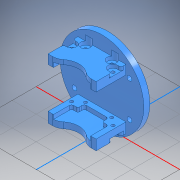
# Autodesk Inventor part: 000.005.005.001 - ОСНОВАНИЕ
Saved by Autodesk Inventor 2022 (Build 260153000, 153)
## iProperties
Created: 2022-12-19
Part Number: 000.005.005.001 - ОСНОВАНИЕ
Material: Пластик АБС
Document SubType Name: Modeling
Designer: Ivan Petrov
Density: 1.06 g/cm^3
Appearance: Голубой
Author: Ivan Petrov
Autodesk Inventor part; units mm, degrees
ref_plane "YZ Plane" through (0, 0, 0) normal (1, 0, 0) x (0, 1, 0)
ref_plane "XZ Plane" through (0, 0, 0) normal (0, 1, 0) x (-1, 0, 0)
ref_plane "XY Plane" through (0, 0, 0) normal (0, 0, 1) x (1, 0, 0)
sketch "Эскиз1" plane through (0, 0, 0) normal (0, 0, 1) x (1, 0, 0)
  circle A0 centre (0, 0) radius 35
  dimension "d7" = 70
  constraints: 1 centre point
  measures "d7" diameter of A0
sketch "Эскиз1 outline for Выдавливание1" plane through (0, 0, 0) normal (0, 0, 1) x (1, 0, 0)
  circle A0 centre (0, 0) radius 35
extrude "Выдавливание1" add sketch "Эскиз1 outline for Выдавливание1" along normal blind 5
sketch "Эскиз2" plane through (0, 0, 5) normal (0, 0, 1) x (1, 0, 0)
  circle A0 centre (-23, 15) radius 2
  point P0 (0, 0)
  dimension "d4" = 4
  dimension "d5" = 15
  dimension "d6" = 23
  constraints: 1 centre point
  measures "d4" diameter of A0
  measures "d5" vertical distance of A0.centre point (0, 0)
  measures "d6" horizontal distance of point (0, 0) A0.centre
sketch "Эскиз2 outline for Выдавливание2" plane through (0, 0, 5) normal (0, 0, 1) x (1, 0, 0)
  circle A0 centre (-23, 15) radius 2
extrude "Выдавливание2" cut sketch "Эскиз2 outline for Выдавливание2" against normal through all
mirror "Зеркальное отражение1" about plane through (0, 0, 0) normal (0, 1, 0) of "Выдавливание2"
mirror "Зеркальное отражение2" about plane through (0, 0, 0) normal (1, 0, 0) of "Выдавливание2", "Зеркальное отражение1"
sketch "Эскиз9" plane through (0, 0, 5) normal (0, 0, 1) x (1, 0, 0)
  line L0 (20.1, 16) -> (20.1, 13.5) projected
  line L1 (-20.1, 16) -> (-20.1, 13.5) projected
  line L2 (20.1, 16) -> (-20.1, 16)
  line L3 (-20.1, 16) -> (-20.1, 18.6)
  line L4 (-20.1, 18.6) -> (20.1, 18.6)
  line L5 (20.1, 18.6) -> (20.1, 16)
  line L6 (-13, 18.6) -> (13, 18.6)
  point P0 (0, 0)
  constraints: 10 end point, 2 horizontal, 2 parallel, 1 perpendicular, 1 point on line, 2 other
sketch "Эскиз9 outline for Выдавливание8" plane through (0, 0, 5) normal (0, 0, 1) x (1, 0, 0)
  line L0 (-20.1, 18.6) -> (-20.1, 16)
  line L1 (20.1, 18.6) -> (-20.1, 18.6)
  line L2 (20.1, 16) -> (20.1, 18.6)
  line L3 (-20.1, 16) -> (20.1, 16)
extrude "Выдавливание8" add sketch "Эскиз9 outline for Выдавливание8" along normal blind 25
sketch "Эскиз10" plane through (0, 0, 5) normal (0, 0, 1) x (1, 0, 0)
  line L0 (20.1, -15.5) -> (20.1, -18)
  line L1 (-20.1, -15.5) -> (-20.1, -18)
  line L2 (20.1, -18) -> (-20.1, -18)
  line L3 (-20.1, -18) -> (-20.1, -21.499996)
  line L4 (-20.1, -21.499996) -> (20.1, -21.499996)
  line L5 (20.1, -21.499996) -> (20.1, -18)
  line L6 (7.682609, -21.499996) -> (-7.682606, -21.5)
  point P0 (0, 0)
  constraints: 8 end point, 2 parallel, 1 horizontal, 1 perpendicular, 1 point on line
sketch "Эскиз10 outline for Выдавливание9" plane through (0, 0, 5) normal (0, 0, 1) x (1, 0, 0)
  line L0 (20.1, -21.499996) -> (20.1, -18)
  line L1 (-20.1, -21.499996) -> (20.1, -21.499996)
  line L2 (-20.1, -18) -> (-20.1, -21.499996)
  line L3 (20.1, -18) -> (-20.1, -18)
extrude "Выдавливание9" add sketch "Эскиз10 outline for Выдавливание9" along normal blind 25
sketch "Эскиз11" plane through (-20.1, 18.6, 5) normal (0, 1, 0) x (1, 0, 0)
  arc A0 (0, -52.676629) -> (0.51922, -54.36356) centre (3, -52.676629) ccw
  line L0 (0.51922, -54.36356) -> (4.504742, -60.22462)
  arc A1 (4.504742, -60.22462) -> (6.158595, -61.1) centre (6.158595, -59.1) ccw
  line L1 (7.1, -61.1) -> (6.158595, -61.1)
  arc A2 (5.6, -59.6) -> (7.1, -61.1) centre (7.1, -59.6) ccw
  line L2 (5.6, -6.6) -> (5.6, -59.6)
  arc A3 (6.6, -5.6) -> (5.6, -6.6) centre (6.6, -6.6) ccw
  line L3 (33.6, -5.6) -> (6.6, -5.6)
  arc A4 (34.6, -6.6) -> (33.6, -5.6) centre (33.6, -6.6) ccw
  line L4 (34.6, -59.6) -> (34.6, -6.6)
  arc A5 (33.1, -61.1) -> (34.6, -59.6) centre (33.1, -59.6) ccw
  line L5 (34.041405, -61.1) -> (33.1, -61.1)
  arc A6 (34.041405, -61.1) -> (35.695258, -60.22462) centre (34.041405, -59.1) ccw
  line L6 (35.695258, -60.22462) -> (39.68078, -54.36356)
  arc A7 (39.68078, -54.36356) -> (40.2, -52.676629) centre (37.2, -52.676629) ccw
  line L7 (40.2, -52.676629) -> (40.2, -8.423371)
  arc A8 (40.2, -8.423371) -> (39.68078, -6.73644) centre (37.2, -8.423371) ccw
  line L8 (39.68078, -6.73644) -> (35.992888, -1.31307)
  arc A9 (35.992888, -1.31307) -> (33.512108, 0) centre (33.512108, -3) ccw
  line L9 (33.512108, 0) -> (6.687892, 0)
  arc A10 (6.687892, 0) -> (4.207112, -1.31307) centre (6.687892, -3) ccw
  line L10 (4.207112, -1.31307) -> (0.51922, -6.73644)
  arc A11 (0.51922, -6.73644) -> (0, -8.423371) centre (3, -8.423371) ccw
  line L11 (0, -8.423371) -> (0, -52.676629)
  circle A12 centre (37.4, -52.1) radius 1.35
  circle A13 centre (37.4, -30.1) radius 1.35
  circle A14 centre (31.1, -2.8) radius 1.35
  circle A15 centre (2.8, -52.1) radius 1.35
  circle A16 centre (2.8, -30.1) radius 1.35
  circle A17 centre (9.1, -2.8) radius 1.35
  circle A18 centre (37.4, -8.1) radius 1.35
  circle A19 centre (2.8, -8.1) radius 1.35
  line L12 (7.1, -61.1) -> (33.1, -61.1)
  point P0 (20.1, 5)
  point P1 (20.1, -48.1)
  point P2 (20.1, -48.1)
  constraints: 26 end point, 24 point on circle, 20 centre point
sketch "Эскиз11 outline for Выдавливание10" plane through (-20.1, 18.6, 5) normal (0, 1, 0) x (1, 0, 0)
  circle A0 centre (2.8, -8.1) radius 1.35
  circle A1 centre (9.1, -2.8) radius 1.35
  circle A2 centre (31.1, -2.8) radius 1.35
  circle A3 centre (37.4, -8.1) radius 1.35
extrude "Выдавливание10" cut sketch "Эскиз11 outline for Выдавливание10" against normal through all
sketch "Эскиз12" plane through (-20.1, 18.6, 5) normal (0, 1, 0) x (1, 0, 0)
  arc A0 (0, -52.676629) -> (0.51922, -54.36356) centre (3, -52.676629) ccw
  line L0 (0.51922, -54.36356) -> (4.504742, -60.22462)
  arc A1 (4.504742, -60.22462) -> (6.158595, -61.1) centre (6.158595, -59.1) ccw
  line L1 (7.1, -61.1) -> (6.158595, -61.1)
  arc A2 (5.6, -59.6) -> (7.1, -61.1) centre (7.1, -59.6) ccw
  line L2 (5.6, -6.6) -> (5.6, -59.6)
  arc A3 (6.6, -5.6) -> (5.6, -6.6) centre (6.6, -6.6) ccw
  line L3 (33.6, -5.6) -> (6.6, -5.6)
  arc A4 (34.6, -6.6) -> (33.6, -5.6) centre (33.6, -6.6) ccw
  line L4 (34.6, -59.6) -> (34.6, -6.6)
  arc A5 (33.1, -61.1) -> (34.6, -59.6) centre (33.1, -59.6) ccw
  line L5 (34.041405, -61.1) -> (33.1, -61.1)
  arc A6 (34.041405, -61.1) -> (35.695258, -60.22462) centre (34.041405, -59.1) ccw
  line L6 (35.695258, -60.22462) -> (39.68078, -54.36356)
  arc A7 (39.68078, -54.36356) -> (40.2, -52.676629) centre (37.2, -52.676629) ccw
  line L7 (40.2, -52.676629) -> (40.2, -8.423371)
  arc A8 (40.2, -8.423371) -> (39.68078, -6.73644) centre (37.2, -8.423371) ccw
  line L8 (39.68078, -6.73644) -> (35.992888, -1.31307)
  arc A9 (35.992888, -1.31307) -> (33.512108, 0) centre (33.512108, -3) ccw
  line L9 (33.512108, 0) -> (6.687892, 0)
  arc A10 (6.687892, 0) -> (4.207112, -1.31307) centre (6.687892, -3) ccw
  line L10 (4.207112, -1.31307) -> (0.51922, -6.73644)
  arc A11 (0.51922, -6.73644) -> (0, -8.423371) centre (3, -8.423371) ccw
  line L11 (0, -8.423371) -> (0, -52.676629)
  circle A12 centre (37.4, -52.1) radius 1.35
  circle A13 centre (37.4, -30.1) radius 1.35
  circle A14 centre (31.1, -2.8) radius 1.35
  circle A15 centre (2.8, -52.1) radius 1.35
  circle A16 centre (2.8, -30.1) radius 1.35
  circle A17 centre (9.1, -2.8) radius 1.35
  circle A18 centre (37.4, -8.1) radius 1.35
  circle A19 centre (2.8, -8.1) radius 1.35
  line L12 (7.1, -61.1) -> (33.1, -61.1)
  point P0 (20.1, 5)
  point P1 (20.1, 5)
  point P2 (20.1, -48.1)
  point P3 (20.1, -48.1)
  constraints: 26 end point, 24 point on circle, 20 centre point
sketch "Эскиз12 outline for Выдавливание11" plane through (-20.1, 18.6, 5) normal (0, 1, 0) x (1, 0, 0)
  line L0 (34.6, -59.6) -> (34.6, -6.6)
  arc A0 (33.1, -61.1) -> (34.6, -59.6) centre (33.1, -59.6) ccw
  line L1 (7.1, -61.1) -> (33.1, -61.1)
  arc A1 (5.6, -59.6) -> (7.1, -61.1) centre (7.1, -59.6) ccw
  line L2 (5.6, -6.6) -> (5.6, -59.6)
  arc A2 (6.6, -5.6) -> (5.6, -6.6) centre (6.6, -6.6) ccw
  line L3 (33.6, -5.6) -> (6.6, -5.6)
  arc A3 (34.6, -6.6) -> (33.6, -5.6) centre (33.6, -6.6) ccw
extrude "Выдавливание11" cut sketch "Эскиз12 outline for Выдавливание11" against normal blind 10
sketch "Эскиз13" plane through (-20.1, -21.499996, 5) normal (0, -1, 0) x (1, 0, 0)
  arc A0 (0.51922, 54.36356) -> (0, 52.676629) centre (3, 52.676629) ccw
  line L0 (0, 8.423371) -> (0, 52.676629)
  arc A1 (0, 8.423371) -> (0.51922, 6.73644) centre (3, 8.423371) ccw
  line L1 (4.207112, 1.31307) -> (0.51922, 6.73644)
  arc A2 (4.207112, 1.31307) -> (6.687892, 0) centre (6.687892, 3) ccw
  line L2 (33.512108, 0) -> (6.687892, 0)
  arc A3 (33.512108, 0) -> (35.992888, 1.31307) centre (33.512108, 3) ccw
  line L3 (39.68078, 6.73644) -> (35.992888, 1.31307)
  arc A4 (39.68078, 6.73644) -> (40.2, 8.423371) centre (37.2, 8.423371) ccw
  line L4 (40.2, 52.676629) -> (40.2, 8.423371)
  arc A5 (40.2, 52.676629) -> (39.68078, 54.36356) centre (37.2, 52.676629) ccw
  line L5 (35.695258, 60.22462) -> (39.68078, 54.36356)
  arc A6 (35.695258, 60.22462) -> (34.041405, 61.1) centre (34.041405, 59.1) ccw
  line L6 (27.75, 61.1) -> (34.041405, 61.1)
  arc A7 (29.25, 59.6) -> (27.75, 61.1) centre (27.75, 59.6) ccw
  line L7 (29.25, 59.6) -> (29.25, 58.1)
  arc A8 (29.25, 58.1) -> (31.6, 55.75) centre (31.6, 58.1) ccw
  line L8 (31.6, 55.75) -> (33.6, 55.75)
  arc A9 (34.6, 54.75) -> (33.6, 55.75) centre (33.6, 54.75) ccw
  line L9 (34.6, 54.75) -> (34.6, 11.95)
  arc A10 (33.6, 10.95) -> (34.6, 11.95) centre (33.6, 11.95) ccw
  line L10 (33.6, 10.95) -> (31.6, 10.95)
  arc A11 (31.6, 10.95) -> (29.25, 8.6) centre (31.6, 8.6) ccw
  line L11 (29.25, 8.6) -> (29.25, 6.6)
  arc A12 (28.25, 5.6) -> (29.25, 6.6) centre (28.25, 6.6) ccw
  line L12 (28.25, 5.6) -> (11.95, 5.6)
  arc A13 (10.95, 6.6) -> (11.95, 5.6) centre (11.95, 6.6) ccw
  line L13 (10.95, 6.6) -> (10.95, 8.6)
  arc A14 (10.95, 8.6) -> (8.6, 10.95) centre (8.6, 8.6) ccw
  line L14 (8.6, 10.95) -> (6.6, 10.95)
  arc A15 (5.6, 11.95) -> (6.6, 10.95) centre (6.6, 11.95) ccw
  line L15 (5.6, 11.95) -> (5.6, 54.75)
  arc A16 (6.6, 55.75) -> (5.6, 54.75) centre (6.6, 54.75) ccw
  line L16 (6.6, 55.75) -> (8.6, 55.75)
  arc A17 (8.6, 55.75) -> (10.95, 58.1) centre (8.6, 58.1) ccw
  line L17 (10.95, 58.1) -> (10.95, 59.6)
  arc A18 (12.45, 61.1) -> (10.95, 59.6) centre (12.45, 59.6) ccw
  line L18 (6.158595, 61.1) -> (12.45, 61.1)
  arc A19 (6.158595, 61.1) -> (4.504742, 60.22462) centre (6.158595, 59.1) ccw
  line L19 (0.51922, 54.36356) -> (4.504742, 60.22462)
  circle A20 centre (37.4, 52.1) radius 1.35
  circle A21 centre (37.4, 30.1) radius 1.35
  circle A22 centre (31.1, 2.8) radius 1.35
  circle A23 centre (2.8, 52.1) radius 1.35
  circle A24 centre (2.8, 30.1) radius 1.35
  circle A25 centre (9.1, 2.8) radius 1.35
  circle A26 centre (37.4, 8.1) radius 1.35
  circle A27 centre (2.8, 8.1) radius 1.35
  circle A28 centre (20.1, 48.1) radius 1.6
  line L20 (12.45, 61.1) -> (27.75, 61.1)
  point P0 (20.1, -5)
  constraints: 42 end point, 40 point on circle, 28 centre point, 1 horizontal
sketch "Эскиз13 outline for Выдавливание12" plane through (-20.1, -21.499996, 5) normal (0, -1, 0) x (1, 0, 0)
  arc A0 (12.45, 61.1) -> (10.95, 59.6) centre (12.45, 59.6) ccw
  line L0 (27.75, 61.1) -> (12.45, 61.1)
  line L1 (10.95, 59.6) -> (10.95, 58.1)
  arc A1 (29.25, 59.6) -> (27.75, 61.1) centre (27.75, 59.6) ccw
  arc A2 (10.95, 58.1) -> (8.6, 55.75) centre (8.6, 58.1) cw
  line L2 (29.25, 58.1) -> (29.25, 59.6)
  line L3 (8.6, 55.75) -> (6.6, 55.75)
  arc A3 (31.6, 55.75) -> (29.25, 58.1) centre (31.6, 58.1) cw
  arc A4 (6.6, 55.75) -> (5.6, 54.75) centre (6.6, 54.75) ccw
  line L4 (33.6, 55.75) -> (31.6, 55.75)
  line L5 (5.6, 54.75) -> (5.6, 11.95)
  arc A5 (34.6, 54.75) -> (33.6, 55.75) centre (33.6, 54.75) ccw
  arc A6 (5.6, 11.95) -> (6.6, 10.95) centre (6.6, 11.95) ccw
  line L6 (34.6, 11.95) -> (34.6, 54.75)
  line L7 (6.6, 10.95) -> (8.6, 10.95)
  arc A7 (33.6, 10.95) -> (34.6, 11.95) centre (33.6, 11.95) ccw
  arc A8 (8.6, 10.95) -> (10.95, 8.6) centre (8.6, 8.6) cw
  line L8 (31.6, 10.95) -> (33.6, 10.95)
  line L9 (10.95, 8.6) -> (10.95, 6.6)
  arc A9 (29.25, 8.6) -> (31.6, 10.95) centre (31.6, 8.6) cw
  arc A10 (10.95, 6.6) -> (11.95, 5.6) centre (11.95, 6.6) ccw
  line L10 (29.25, 6.6) -> (29.25, 8.6)
  line L11 (11.95, 5.6) -> (28.25, 5.6)
  arc A11 (28.25, 5.6) -> (29.25, 6.6) centre (28.25, 6.6) ccw
  circle A12 centre (20.1, 48.1) radius 1.6
extrude "Выдавливание12" cut sketch "Эскиз13 outline for Выдавливание12" against normal blind 10
offset faces "Размер5" outward -1 faces at (-14.5, 17.733333, 17.733333) (-14.455573, 17.733333, 11.305245) (4.5, 17.733333, 10.6) (14.430874, 16.866667, 11.234659) (14.5, 17.733333, 23.866667) (-2.716667, -20.333331, 10.6) (8.22473, -20.333331, 10.602796) (9.176248, -19.166665, 13.950249) (9.15, -20.333331, 12.266667) (12.166667, -20.333331, 15.95) (14.488831, -19.166665, 16.800958) (14.5, -19.166665, 21.3) (-9.138831, -19.166665, 11.450958) (-9.15, -20.333331, 12.933333) (-11.149751, -19.166665, 15.923752) (-12.833333, -19.166665, 15.95) (-14.180173, -19.166665, 16.216948) (-14.5, -20.333331, 25.65)
sketch "Эскиз14" plane through (-20.1, -21.499996, 5) normal (0, -1, 0) x (1, 0, 0)
  line L0 (35.6, 25) -> (35.6, 11.95) projected
  arc A0 (33.6, 9.95) -> (35.6, 11.95) centre (33.6, 11.95) ccw projected
  line L1 (33.6, 9.95) -> (31.6, 9.95) projected
  arc A1 (31.6, 9.95) -> (30.25, 8.6) centre (31.6, 8.6) ccw projected
  line L2 (30.25, 8.6) -> (30.25, 6.6) projected
  arc A2 (28.25, 4.6) -> (30.25, 6.6) centre (28.25, 6.6) ccw projected
  line L3 (28.25, 4.6) -> (11.95, 4.6) projected
  arc A3 (9.95, 6.6) -> (11.95, 4.6) centre (11.95, 6.6) ccw projected
  line L4 (9.95, 6.6) -> (9.95, 8.6) projected
  arc A4 (9.95, 8.6) -> (8.6, 9.95) centre (8.6, 8.6) ccw projected
  line L5 (8.6, 9.95) -> (6.6, 9.95) projected
  arc A5 (4.6, 11.95) -> (6.6, 9.95) centre (6.6, 11.95) ccw projected
  line L6 (4.6, 11.95) -> (4.6, 25) projected
  line L7 (0, 25) -> (4.6, 25) projected
  line L8 (0, 0) -> (0, 25) projected
  line L9 (40.2, 0) -> (0, 0) projected
  line L10 (40.2, 0) -> (40.2, 25) projected
  line L11 (35.6, 25) -> (40.2, 25) projected
  circle A6 centre (37.4, 8.1) radius 1.35 projected
  circle A7 centre (2.8, 8.1) radius 1.35 projected
  circle A8 centre (31.1, 2.8) radius 1.35 projected
  circle A9 centre (9.1, 2.8) radius 1.35 projected
  line L12 (4.6, 6.6) -> (4.6, 25) projected
  line L13 (4.6, 25) -> (36.05, 25)
  point P0 (20.1, -5)
  constraints: 2 end point, 1 point on line
sketch "Эскиз14 outline for Выдавливание13" plane through (-20.1, -21.499996, 5) normal (0, -1, 0) x (1, 0, 0)
  line L0 (4.6, 25) -> (0, 25)
  line L1 (35.6, 25) -> (4.6, 25)
  line L2 (0, 25) -> (0, 0)
  line L3 (40.2, 25) -> (35.6, 25)
  line L4 (0, 0) -> (40.2, 0)
  line L5 (40.2, 0) -> (40.2, 25)
  circle A0 centre (9.1, 2.8) radius 1.35
  circle A1 centre (31.1, 2.8) radius 1.35
  circle A2 centre (2.8, 8.1) radius 1.35
  circle A3 centre (37.4, 8.1) radius 1.35
extrude "Выдавливание13" add sketch "Эскиз14 outline for Выдавливание13" along normal blind 5
sketch "Эскиз15" plane through (-20.1, 18.6, 5) normal (0, 1, 0) x (1, 0, 0)
  line L0 (4.6, -25) -> (4.6, -6.6) projected
  arc A0 (6.6, -4.6) -> (4.6, -6.6) centre (6.6, -6.6) ccw projected
  line L1 (6.6, -4.6) -> (33.6, -4.6) projected
  arc A1 (35.6, -6.6) -> (33.6, -4.6) centre (33.6, -6.6) ccw projected
  line L2 (35.6, -6.6) -> (35.6, -25) projected
  line L3 (40.2, -25) -> (35.6, -25) projected
  line L4 (40.2, 0) -> (40.2, -25) projected
  line L5 (0, 0) -> (40.2, 0) projected
  line L6 (0, 0) -> (0, -25) projected
  line L7 (4.6, -25) -> (0, -25) projected
  circle A2 centre (37.4, -8.1) radius 1.35 projected
  circle A3 centre (2.8, -8.1) radius 1.35 projected
  circle A4 centre (31.1, -2.8) radius 1.35 projected
  circle A5 centre (9.1, -2.8) radius 1.35 projected
  line L8 (35.6, -25) -> (4.6, -25)
  line L9 (40.2, -25) -> (0, -25) projected
  point P0 (20.1, 5)
  constraints: 2 end point, 1 collinear
sketch "Эскиз15 outline for Выдавливание14" plane through (-20.1, 18.6, 5) normal (0, 1, 0) x (1, 0, 0)
  line L0 (4.6, -25) -> (35.6, -25)
  line L1 (0, -25) -> (4.6, -25)
  line L2 (35.6, -25) -> (40.2, -25)
  line L3 (0, 0) -> (0, -25)
  line L4 (40.2, -25) -> (40.2, 0)
  line L5 (40.2, 0) -> (0, 0)
  circle A0 centre (2.8, -8.1) radius 1.35
  circle A1 centre (37.4, -8.1) radius 1.35
  circle A2 centre (9.1, -2.8) radius 1.35
  circle A3 centre (31.1, -2.8) radius 1.35
extrude "Выдавливание14" add sketch "Эскиз15 outline for Выдавливание14" along normal blind 5
sketch "Эскиз16" plane through (-20.1, 23.6, 5) normal (0, 1, 0) x (1, 0, 0)
  circle A0 centre (37.4, -8.1) radius 1.35 projected
  circle A1 centre (37.4, -8.1) radius 4
  circle A2 centre (31.1, -2.8) radius 1.35 projected
  circle A3 centre (31.1, -2.8) radius 4
  circle A4 centre (2.8, -8.1) radius 1.35 projected
  circle A5 centre (2.8, -8.1) radius 4
  circle A6 centre (9.1, -2.8) radius 1.35 projected
  circle A7 centre (9.1, -2.8) radius 4
  point P0 (20.1, 5)
  dimension "d51" = 8
  dimension "d52" = 8
  dimension "d53" = 8
  dimension "d54" = 8
  constraints: 4 centre point, 4 coincident
  measures "d51" diameter of A1
  measures "d52" diameter of A3
  measures "d53" diameter of A5
  measures "d54" diameter of A7
sketch "Эскиз16 outline for Выдавливание15" plane through (-20.1, 23.6, 5) normal (0, 1, 0) x (1, 0, 0)
  circle A0 centre (37.4, -8.1) radius 4
  circle A1 centre (2.8, -8.1) radius 4
  circle A2 centre (31.1, -2.8) radius 4
  circle A3 centre (9.1, -2.8) radius 4
extrude "Выдавливание15" cut sketch "Эскиз16 outline for Выдавливание15" along normal blind 4.5 and the other way blind 3
fillet "Сопряжение3" radius 2 4 edges at (20.1, 22.1, 10.2434) (20.1, 22.1, 15.9566) (-20.1, 22.1, 15.9566) (-20.1, 22.1, 10.2434)
sketch "Эскиз17" plane through (-20.1, -26.499996, 5) normal (0, -1, 0) x (1, 0, 0)
  circle A0 centre (2.8, 8.1) radius 1.35 projected
  circle A1 centre (2.8, 8.1) radius 4
  circle A2 centre (9.1, 2.8) radius 1.35 projected
  circle A3 centre (9.1, 2.8) radius 4
  circle A4 centre (31.1, 2.8) radius 1.35 projected
  circle A5 centre (31.1, 2.8) radius 4
  circle A6 centre (37.4, 8.1) radius 1.35 projected
  circle A7 centre (37.4, 8.1) radius 4
  point P0 (20.1, -5)
  dimension "d60" = 8
  dimension "d61" = 8
  dimension "d62" = 8
  dimension "d63" = 8
  constraints: 4 centre point, 4 coincident
  measures "d60" diameter of A1
  measures "d61" diameter of A3
  measures "d62" diameter of A5
  measures "d63" diameter of A7
sketch "Эскиз17 outline for Выдавливание16" plane through (-20.1, -26.499996, 5) normal (0, -1, 0) x (1, 0, 0)
  circle A0 centre (2.8, 8.1) radius 4
  circle A1 centre (31.1, 2.8) radius 4
  circle A2 centre (9.1, 2.8) radius 4
  circle A3 centre (37.4, 8.1) radius 4
extrude "Выдавливание16" cut sketch "Эскиз17 outline for Выдавливание16" along normal blind 4.5 and the other way blind 3
fillet "Сопряжение4" radius 2 4 edges at (20.1, -25, 15.9566) (20.1, -25, 10.2434) (-20.1, -25, 10.2434) (-20.1, -25, 15.9566)
sketch "Эскиз18" plane through (-20.1, 23.6, 5) normal (0, 1, 0) x (1, 0, 0)
  line L0 (35.6, -25) -> (4.6, -25)
  arc A0 (31.991596, -25) -> (8.208404, -25) centre (20.1, -34.538809) ccw
  line L1 (20.1, 5) -> (20.1, -9.201473) construction
  constraints: 2 end point, 2 point on circle, 2 point on line, 1 centre point, 1 symmetric about line, 1 vertical, 1 vertical alignment
sketch "Эскиз18 outline for Выдавливание17" plane through (-20.1, 23.6, 5) normal (0, 1, 0) x (1, 0, 0)
  arc A0 (31.991596, -25) -> (8.208404, -25) centre (20.1, -34.538809) ccw
  line L0 (8.208404, -25) -> (31.991596, -25)
extrude "Выдавливание17" cut sketch "Эскиз18 outline for Выдавливание17" against normal through all
fillet "Сопряжение5" radius 10.75 4 edges at (11.8916, 21.1, 30) (-11.8916, 21.1, 30) (-11.8916, -24, 30) (11.8916, -24, 30)
move faces "Перенос2" translate (0, 1.3, 0) faces at (0, 18.6, 14.498058)
